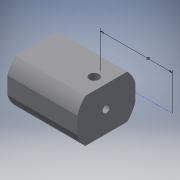
# Autodesk Inventor part: motor_quick
Saved by Autodesk Inventor 2017.2 (Build 212233000, 233)
## iProperties
Created: 2017-07-13
Part Number: motor_quick
Material: Generic
Document SubType Name: Modeling
Designer: Nic
Density: 1 g/cm^3
Appearance: Default
Author: Nic
Autodesk Inventor part; units mm, degrees
ref_plane "YZ Plane" through (0, 0, 0) normal (1, 0, 0) x (0, 1, 0)
ref_plane "XZ Plane" through (0, 0, 0) normal (0, 1, 0) x (-1, 0, 0)
ref_plane "XY Plane" through (0, 0, 0) normal (0, 0, 1) x (1, 0, 0)
sketch "Sketch1" plane through (0, 0, 0) normal (0, 1, 0) x (-1, 0, 0)
  line L0 (14, 9) -> (-14, 9)
  line L1 (-14, 9) -> (-14, -9)
  line L2 (-14, -9) -> (14, -9)
  line L3 (14, -9) -> (14, 9)
  line L4 (0, 0) -> (0, -9) construction
  line L5 (0, 0) -> (-14, 0) construction
  dimension "d0" = 18
  dimension "d1" = 28
  constraints: 12 end point, 2 midpoint, 2 parallel, 2 perpendicular, 1 horizontal, 1 vertical, 1 other
  measures "d0" distance of L2.end L0.start
  measures "d1" distance of L1.end L2.end
extrude "Extrusion1" add sketch "Sketch1" along normal blind 24
sketch "Sketch4" plane through (-14, 0, 9) normal (0, 0, 1) x (1, 0, 0)
  line L0 (0, 0) -> (0, 24) construction
  line L1 (0, 12) -> (31.0841, 12) construction
  circle A0 centre (23, 12) radius 2
  line L2 (28, 0) -> (28, 24) projected
  point P0 (14, 0)
  dimension "d4" = 4
  dimension "d5" = 5
  constraints: 2 end point, 1 centre point, 1 horizontal, 1 midpoint, 1 point on line
  measures "d4" diameter of A0
  measures "d5" distance from line of L2 A0.centre
extrude "Extrusion2" cut sketch "Sketch4" against normal up to next
sketch "Sketch5" plane through (14, 0, 9) normal (1, 0, 0) x (0, 0, -1)
  circle A0 centre (9, 12) radius 1.5
  line L0 (0, 0) -> (0, 24) construction
  line L1 (0, 12) -> (9.7328, 12) construction
  line L2 (9, 0) -> (9, 12) construction
  circle A1 centre (9, 12) radius 12.5
  circle A2 centre (9, 12) radius 15
  dimension "d8" = 3
  dimension "d9" = 25
  dimension "d10" = 30
  constraints: 4 end point, 3 centre point, 2 coincident, 1 horizontal, 1 midpoint, 1 point on line, 1 vertical
  measures "d8" diameter of A0
  measures "d9" diameter of A1
  measures "d10" diameter of A2
extrude "Extrusion3" cut sketch "Sketch5" against normal up to next
sketch "Sketch6" plane through (0, 24, 0) normal (0, 1, 0) x (1, 0, 0)
  line L0 (0, 0) -> (30, 0) construction
  dimension "d13" = 30
  constraints: 2 end point, 1 horizontal
  measures "d13" distance of L0.start L0.end
body "Solid1"
